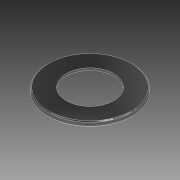
# Autodesk Inventor part: VersaRoller Flange (WCP-0444)
Saved by Autodesk Inventor 2022 (Build 260153000, 153)
## iProperties
Created: 2022-01-25
Part Number: VersaRoller Flange (WCP-0444)
Material: Aluminum 6061
Document SubType Name: Modeling
Designer: Desktop
Density: 2.7 g/cm^3
Appearance: Glazed - Black
Author: Desktop
Autodesk Inventor part; units mm, degrees
ref_plane "YZ Plane" through (0, 0, 0) normal (1, 0, 0) x (0, 1, 0)
ref_plane "XZ Plane" through (0, 0, 0) normal (0, 1, 0) x (-1, 0, 0)
ref_plane "XY Plane" through (0, 0, 0) normal (0, 0, 1) x (1, 0, 0)
sketch "Sketch1" plane through (0, 0, 0) normal (0, 0, 1) x (1, 0, 0)
  line L0 (-24.9, 0) -> (-25.4, 0.5)
  line L1 (-16.6687, 0) -> (-24.9, 0)
  line L2 (-16.6687, 1.5875) -> (-16.6687, 0)
  line L3 (-14.3002, 1.5875) -> (-16.6687, 1.5875)
  line L4 (-14.3002, 3) -> (-14.3002, 1.5875)
  line L5 (-24.9, 3) -> (-14.3002, 3)
  line L6 (-25.4, 2.5) -> (-24.9, 3)
  line L7 (-25.4, 0.5) -> (-25.4, 2.5)
  line L8 (0, 0) -> (0, 6.8981)
  dimension "d0" = 50.8
  dimension "d1" = 28.6004
  dimension "d2" = 3
  dimension "d3" = 1.5875
  dimension "d4" = 2.3685
  dimension "d5" = 0.5
  dimension "d6" = 0.5
  dimension "d7" = 0.5
  dimension "d9" = 0.5
  constraints: 18 end point, 3 perpendicular, 1 coincident, 1 vertical
  measures "d0" diameter of L7 L8
  measures "d1" diameter of L4 L8
  measures "d2" distance between parallel lines of L1 L5
  measures "d3" distance between parallel lines of L1 L3
  measures "d4" distance of L3.start L2.start
  measures "d5" horizontal distance of L6.start L5.start
  measures "d6" horizontal distance of L5.start L6.start
  measures "d7" vertical distance of point (0, 0) L0.end
  measures "d9" horizontal distance of L0.start L0.end
revolve "Revolution1" add sketch "Sketch1" angle 360 about axis through (0, 0, 0) along (0, 1, 0)
equation "\"d6\" = d5"
equation "\"d7\" = d6"
equation "\"d9\" = d7"
body "Solid1"
